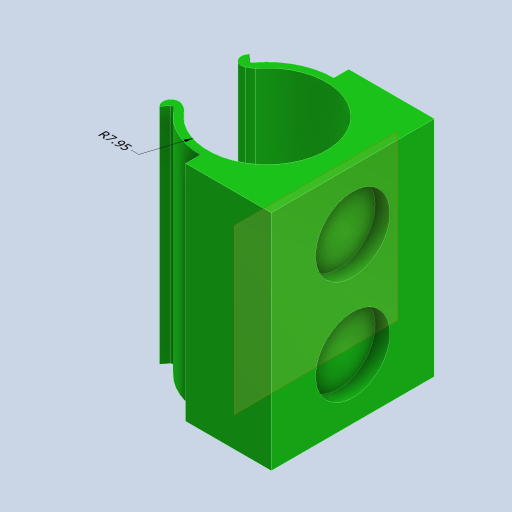
# Autodesk Inventor part: крепление маркера 16мм
Saved by Autodesk Inventor 2024.2 (Build 282272000, 272)
## iProperties
Created: 2025-12-12
Part Number: крепление маркера 16мм
Material: Типовые
Document SubType Name: Modeling
Designer: katya_notebook
Density: 1 g/cm^3
Appearance: Темно-зеленый
Author: katya_notebook
Autodesk Inventor part; units mm, degrees
ref_plane "YZ Plane" through (0, 0, 0) normal (1, 0, 0) x (0, 1, 0)
ref_plane "XZ Plane" through (0, 0, 0) normal (0, 1, 0) x (-1, 0, 0)
ref_plane "XY Plane" through (0, 0, 0) normal (0, 0, 1) x (1, 0, 0)
sketch "Эскиз1" plane through (0, 0, 0) normal (0, 1, 0) x (-1, 0, 0)
  circle A0 centre (0, 0) radius 7.95
  circle A1 centre (0, 0) radius 8.95
  line L0 (0, 0) -> (7.1419, 5.394)
  line L1 (0, 0) -> (7.1419, -5.394)
  point P0 (6.3439, -4.7913)
  point P1 (6.3439, 4.7913)
  dimension "d0" = 15.9
  dimension "d1" = 17.9
  constraints: 4 end point, 2 centre point, 2 coincident, 2 point on circle
  measures "d0" diameter of A0
  measures "d1" diameter of A1
extrude "Выдавливание1" add sketch "Эскиз1" along normal blind 30 contours A0 L1 A1 L0 picked at (-8.5243, 0.7366)
sketch "Эскиз2" plane through (0, 30, 0) normal (0, 1, 0) x (1, 0, 0)
  arc A0 (-6.3439, -4.7913) -> (-7.2366, -4.2614) centre (-9.0453, -8.3253) ccw
  arc A1 (-7.2366, -4.2614) -> (-8.3936, -6.0672) centre (-7.671, -5.2567) ccw
  line L0 (-8.3936, -6.0672) -> (-7.7223, -5.2127)
  arc A2 (-7.1433, -5.3795) -> (-7.7223, -5.2127) centre (-7.5117, -5.5699) ccw
  line L1 (-6.3439, -4.7913) -> (-7.1419, -5.394)
  line L2 (-7.1419, -5.394) -> (-6.3439, -4.7913)
  line L3 (-7.1419, -5.394) -> (-7.1433, -5.3795)
  line L4 (-0.0151, 0) -> (-3.489, 0)
  arc A3 (-7.2366, 4.2614) -> (-6.3439, 4.7913) centre (-9.0453, 8.3253) ccw
  arc A4 (-7.7223, 5.2127) -> (-7.1433, 5.3795) centre (-7.5117, 5.5699) ccw
  line L5 (-6.3439, 4.7913) -> (-7.1419, 5.394)
  line L6 (-7.1419, 5.394) -> (-6.3439, 4.7913)
  line L7 (-7.1419, 5.394) -> (-7.1433, 5.3795)
  arc A5 (-8.3936, 6.0672) -> (-7.2366, 4.2614) centre (-7.671, 5.2567) ccw
  line L8 (-8.3936, 6.0672) -> (-7.7223, 5.2127)
  point P0 (-6.3439, 4.7913)
  point P1 (-7.1419, -5.394)
  point P2 (-5.3694, -4.0591)
  point P3 (-7.1419, 5.394)
  point P4 (-5.3694, 4.0591)
  point P5 (-7.1419, 5.394)
  dimension "d25" = 1.0859
  constraints: 18 end point, 12 point on circle, 12 symmetric about line, 6 centre point, 4 coincident, 1 collinear, 1 horizontal, 3 other
  measures "d25" radius of A1
sketch "Эскиз3" plane through (0, 30, 0) normal (0, 1, 0) x (1, 0, 0)
  arc A0 (-7.1419, -5.394) -> (-7.1419, 5.394) centre (0, 0) ccw projected
  line L0 (11.5, -6.95) -> (11.5, 6.95)
  arc A1 (-6.3439, -4.7913) -> (-6.3439, 4.7913) centre (0, 0) ccw projected
  arc A2 (0, -7.95) -> (0, 7.95) centre (2.8636, 0) ccw
  line L1 (0, -8.95) -> (0, -7.95)
  line L2 (0, 7.95) -> (0, 8.95)
  line L3 (11.5, 6.95) -> (11.5, 10.95)
  line L4 (11.5, -6.95) -> (11.5, -10.95)
  line L5 (0, 4.45) -> (0, 8.95)
  line L6 (11.5, -10.95) -> (0, -10.95)
  line L7 (0, -10.95) -> (0, -8.95)
  line L8 (11.5, 10.95) -> (0, 10.95)
  line L9 (0, 10.95) -> (0, 8.95)
  point P0 (0, 7.95)
  dimension "d13" = 4
  dimension "d14" = 4
  dimension "d22" = 21.9
  dimension "d23" = 3
  constraints: 20 end point, 6 point on circle, 4 vertical, 2 horizontal, 2 perpendicular, 1 centre point, 1 collinear
  measures "d13" distance of L4.end L0.start
  measures "d14" distance of L3.end L0.end
  measures "d22" distance of L4.end L3.end
  measures "d23" distance of L6.end L1.end
extrude "Выдавливание3" add sketch "Эскиз3" against normal blind 30 contours L1 A2 A0 | A0 A2 L9 L8 L3 L0 L4 L6 L7 | A2 L2 A0
ref_plane "РабПлоскость1" through (11.5, 20, 4.95) normal (1, 0, 0) x (0, 0, -1)
sketch "Эскиз4" plane through (11.5, 20, 4.95) normal (1, 0, 0) x (0, 0, -1)
  line L0 (4.95, -20) -> (4.95, 10)
  line L1 (1, 10) -> (8.9, 10) projected
  circle A0 centre (4.95, -12) radius 5
  line L2 (14.4, -20) -> (-4.5, -20) projected
  circle A1 centre (4.95, 2) radius 5
  line L3 (-4.5, 10) -> (14.4, 10) projected
  point P0 (7.3306, 10)
  point P1 (2.5694, 10)
  point P2 (4.95, 10)
  dimension "d15" = 10
  dimension "d16" = 8
  dimension "d17" = 10
  dimension "d18" = 8
  constraints: 3 midpoint, 2 centre point, 2 end point, 2 point on line
  measures "d15" diameter of A0
  measures "d16" distance of A0.centre point (4.95, -20)
  measures "d17" diameter of A1
  measures "d18" distance of point (4.95, 10) A1.centre
extrude "Выдавливание4" cut sketch "Эскиз4" against normal blind 2
extrude "Выдавливание5" add sketch "Эскиз2" against normal blind 30
sketch "Эскиз5" plane through (0, 30, 0) normal (0, 1, 0) x (1, 0, 0)
  arc A0 (0, 8.95) -> (-7.1419, 5.394) centre (0, 0) ccw projected
  line L0 (-7.1419, 5.394) -> (-7.1433, 5.3795) projected
  arc A1 (-7.7223, 5.2127) -> (-7.1433, 5.3795) centre (-7.5117, 5.5699) ccw projected
  line L1 (-7.7223, 5.2127) -> (-8.3936, 6.0672) projected
  arc A2 (-8.3936, 6.0672) -> (-7.2366, 4.2614) centre (-7.671, 5.2567) ccw projected
  arc A3 (-7.2366, 4.2614) -> (-6.3439, 4.7913) centre (-9.0453, 8.3253) ccw projected
  arc A4 (-6.3439, -4.7913) -> (-6.3439, 4.7913) centre (0, 0) ccw projected
  arc A5 (-6.3439, -4.7913) -> (-7.2366, -4.2614) centre (-9.0453, -8.3253) ccw projected
  arc A6 (-7.2366, -4.2614) -> (-8.3936, -6.0672) centre (-7.671, -5.2567) ccw projected
  line L2 (-8.3936, -6.0672) -> (-7.7223, -5.2127) projected
  arc A7 (-7.1433, -5.3795) -> (-7.7223, -5.2127) centre (-7.5117, -5.5699) ccw projected
  line L3 (-7.1433, -5.3795) -> (-7.1419, -5.394) projected
  arc A8 (-7.1419, -5.394) -> (0, -8.95) centre (0, 0) ccw projected
  line L4 (0, -8.95) -> (0, -10.95) projected
  line L5 (0, -10.95) -> (11.5, -10.95) projected
  line L6 (11.5, -10.95) -> (11.5, 10.95) projected
  line L7 (11.5, 10.95) -> (0, 10.95) projected
  line L8 (0, 10.95) -> (0, 8.95) projected
  arc A9 (2.9509, -8.4495) -> (2.9509, 8.4495) centre (2.8636, 0) ccw projected
  arc A10 (2.9509, -8.4495) -> (2.9509, 8.4495) centre (0, 0) ccw projected
  line L9 (0, 7.95) -> (0, 8.95)
  line L10 (0, -7.95) -> (0, -8.95)
  constraints: 4 end point, 2 point on circle, 1 collinear, 1 point on line, 1 vertical
extrude "Выдавливание6" add sketch "Эскиз5" against normal blind 30 contours A10 A9
sketch "Эскиз6" plane through (11.5, 30, 10.95) normal (1, 0, 0) x (0, 0, -1)
  circle A0 centre (10.95, -22) radius 5 projected
  circle A1 centre (10.95, -8) radius 5 projected
  point P0 (10.95, -30)
extrude "Выдавливание7" cut sketch "Эскиз6" against normal blind 2
